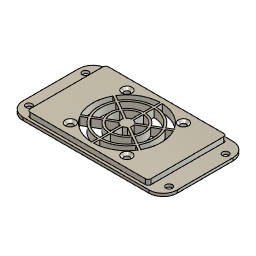
LCD cooling fan mod (Autodesk Fusion 360 design; units mm, degrees)
Autodesk Fusion 360 part; units mm, degrees
sketch "Sketch1" plane through (0, 0, 0) normal (0, 1, 0) x (1, 0, 0)
  line L0 (0, 0) -> (85.6, 0)
  line L1 (85.6, 0) -> (85.6, 55.5)
  line L2 (85.6, 55.5) -> (0, 55.5)
  line L3 (0, 55.5) -> (0, 0)
  line L4 (0, 55.5) -> (85.6, 0) construction
  line L5 (0, 0) -> (85.6, 55.5) construction
  line L6 (62.8, 47.75) -> (22.8, 47.75) construction
  line L7 (22.8, 47.75) -> (22.8, 7.75) construction
  line L8 (22.8, 7.75) -> (62.8, 7.75) construction
  line L9 (62.8, 7.75) -> (62.8, 47.75) construction
  line L10 (62.8, 47.75) -> (22.8, 7.75) construction
  line L11 (22.8, 47.75) -> (62.8, 7.75) construction
  circle A0 centre (62.8, 47.75) radius 1.9
  circle A1 centre (62.8, 7.75) radius 1.9
  circle A2 centre (22.8, 7.75) radius 1.9
  circle A3 centre (22.8, 47.75) radius 1.9
  line L12 (68.05, 2.5) -> (17.55, 2.5) construction
  line L13 (17.55, 2.5) -> (17.55, 53) construction
  line L14 (17.55, 53) -> (68.05, 53) construction
  line L15 (68.05, 53) -> (68.05, 2.5) construction
  line L16 (68.05, 2.5) -> (17.55, 53) construction
  line L17 (17.55, 2.5) -> (68.05, 53) construction
  circle A4 centre (42.8, 27.75) radius 24.25
  line L18 (43.55, 53) -> (42.05, 53) construction
  line L19 (42.05, 53) -> (42.05, 27.75)
  line L20 (42.05, 27.75) -> (43.55, 27.75)
  line L21 (43.55, 27.75) -> (43.55, 53)
  line L22 (43.175, 28.3995) -> (21.3079, 41.0245)
  line L23 (20.5579, 39.7255) -> (42.425, 27.1005)
  line L24 (42.425, 28.3995) -> (20.5579, 15.7745)
  line L25 (21.3079, 14.4755) -> (43.175, 27.1005)
  line L26 (42.05, 27.75) -> (42.05, 2.5)
  line L27 (43.55, 2.5) -> (43.55, 27.75)
  line L28 (42.425, 27.1005) -> (64.2921, 14.4755)
  line L29 (65.0421, 15.7745) -> (43.175, 28.3995)
  line L30 (43.175, 27.1005) -> (65.0421, 39.7255)
  line L31 (64.2921, 41.0245) -> (42.425, 28.3995)
  circle A5 centre (42.8, 27.75) radius 20
  circle A6 centre (42.8, 27.75) radius 18.5
  circle A7 centre (42.8, 27.75) radius 12.5
  circle A8 centre (42.8, 27.75) radius 11
  circle A9 centre (42.8, 27.75) radius 4
  line L32 (85.6, 7.25) -> (95.4, 7.25) construction
  circle A10 centre (93.15, 7.25) radius 2.25
  line L33 (93.15, 7.25) -> (93.15, 9.5) construction
  line L34 (93.15, 9.5) -> (93.15, 45) construction
  circle A11 centre (93.15, 47.25) radius 2.25
  line L35 (93.15, 47.25) -> (93.15, 45) construction
  line L36 (85.6, 0) -> (93.15, 0) construction
  line L37 (93.15, 0) -> (93.15, 7.25) construction
  line L38 (85.6, 7.25) -> (0, 7.25) construction
  line L39 (0, 7.25) -> (-6, 7.25) construction
  line L40 (-6, 7.25) -> (-6, 47.25) construction
  line L41 (93.15, 47.25) -> (-6, 47.25) construction
  circle A12 centre (-6, 47.25) radius 2.25
  circle A13 centre (-6, 7.25) radius 2.25
  line L42 (-11, 57.5) -> (98.15, 57.5)
  line L43 (98.15, 57.5) -> (98.15, -2)
  line L44 (98.15, -2) -> (-11, -2)
  line L45 (-11, -2) -> (-11, 57.5)
  point P0 (42.8, 27.75)
  point P1 (42.8, 27.75)
  dimension "d1" = 85.6
  dimension "d2" = 55.5
  dimension "d3" = 40
  dimension "d4" = 40
  dimension "d5" = 3.8
  dimension "d6" = 3.8
  dimension "d7" = 3.8
  dimension "d8" = 3.8
  dimension "d9" = 50.5
  dimension "d10" = 50.5
  dimension "d11" = 48.5
  dimension "d12" = 1.5
  dimension "d14" = 360
  dimension "d15" = -1.5
  dimension "d16" = 25
  dimension "d17" = -1.5
  dimension "d18" = 8
  dimension "d19" = 9.8
  dimension "d20" = 4.5
  dimension "d21" = 35.5
  dimension "d22" = 4.5
  dimension "d23" = 7.25
  dimension "d24" = 6
  dimension "d25" = 4.5
  dimension "d26" = 4.5
  dimension "d27" = 5
  dimension "d28" = 5
  dimension "d29" = 2
  dimension "d30" = 2
  constraint horizontal L0
  constraint vertical L1
  constraint horizontal L2
  constraint vertical L3
  constraint coincident L0.start L3.end
  constraint horizontal L6
  constraint perpendicular L6 L7
  constraint parallel L6 L8
  constraint parallel L7 L9
  constraint coincident L10 P1
  constraint coincident L11 P1
  constraint midpoint L5 P1
  constraint coincident L6.start L9.end
  constraint coincident L8.end L9.start
  constraint coincident L7.end L8.start
  constraint coincident L6.end L7.start
  constraint horizontal L12
  constraint perpendicular L12 L13
  constraint parallel L12 L14
  constraint parallel L13 L15
  constraint coincident L16 P1
  constraint coincident L17 P1
  constraint coincident P1 P0
  constraint horizontal L18
  constraint vertical L19
  constraint horizontal L20
  constraint vertical L21
  constraint midpoint L14 L18
  constraint midpoint P1 L20
  constraint tangent L9 A5
  constraint concentric A5 A9
  constraint coincident L1 L32.start
  constraint perpendicular L1 L32
  constraint coincident L32.end A10
  constraint coincident A10.centre L33.start
  constraint coincident A10 L33.end
  constraint perpendicular L32 L33
  constraint perpendicular L32 L34
  constraint coincident A11.centre L35.start
  constraint coincident A11 L34.end
  constraint vertical L35
  constraint coincident L34.end L35.end
  constraint coincident L32 A10.centre
  constraint perpendicular L1 L36
  constraint perpendicular L32 L37
  constraint coincident L3 L38.end
  constraint perpendicular L3 L38
  constraint perpendicular L3 L39
  constraint perpendicular L39 L40
  constraint perpendicular L35 L41
  constraint coincident L40 L41.end
  constraint coincident L40.end L41.end
  constraint coincident L39.end L40.start
  constraint horizontal L42
  constraint vertical L43
  constraint horizontal L44
  constraint vertical L45
  measures "d1" distance of L0.start L0.end
  measures "d2" distance of L0.start L2.end
  measures "d3" distance of L7.end L8.end
  measures "d4" distance of L6.end L7.end
  measures "d5" diameter of A0
  measures "d6" diameter of A1
  measures "d7" diameter of A2
  measures "d8" diameter of A3
  measures "d9" distance of L13.end L14.end
  measures "d10" distance of L12.end L13.end
  measures "d11" diameter of A4
  measures "d12" distance of L18.start L18.end
  measures "d16" diameter of A7
  measures "d18" diameter of A9
  measures "d19" distance of L32.start L32.end
  measures "d20" diameter of A10
  measures "d21" distance of L33.end L34.end
  measures "d22" diameter of A11
  measures "d23" distance of L36.end A10.centre
  measures "d24" distance of L38.end L39.end
  measures "d25" diameter of A12
  measures "d26" diameter of A13
  measures "d27" distance of L40.end L45
  measures "d28" distance of A11.centre L43
  measures "d29" distance of L2 L42
  measures "d30" distance of L0 L44
extrude "Extrude1" add sketch "Sketch1" along normal blind 3.6 and the other way blind 2 contours L0 L1 L2 L3 | A4 L30 L31 A5 | A4 L28 L29 A5 | L29 L30 A5 A6 | L30 L31 A5 A6 | L28 L29 A5 A6 | A4 L19 L21 A5 | L21 L31 A5 A6 | L30 L31 A6 A7 | A4 L26 L27 A5 | L27 L28 A5 A6 | L28 L29 A6 A7 | L19 L21 A5 A6 | L29 L30 A7 A8 | L30 L31 A7 A8 | L26 L27 A5 A6 | L28 L29 A7 A8 | A4 L22 L23 A5 | L19 L22 A5 A6 | L19 L21 A6 A7 | L21 L31 A7 A8 | L30 L31 A8 A9 | A4 L24 L25 A5 | L25 L26 A5 A6 | L26 L27 A6 A7 | L27 L28 A7 A8 | L28 L29 A8 A9 | L22 L23 A5 A6 | L19 L21 A7 A8 | L29 L30 A9 | L21 L29 L30 L31 A9 | L24 L25 A5 A6 | L26 L27 A7 A8 | L27 L28 L29 L30 A9 | L23 L24 A5 A6 | L22 L23 A6 A7 | L19 L22 A7 A8 | L19 L21 A8 A9 | L21 L31 A9 | L21 L27 L29 L30 | L24 L25 A6 A7 | L25 L26 A7 A8 | L26 L27 A8 A9 | L27 L28 A9 | L22 L23 A7 A8 | L19 L21 L22 L31 A9 | L21 L22 L29 L31 | L19 L20 L21 L22 L24 L29 L31 | L20 L23 L25 L26 L27 L28 L30 | L25 L27 L28 L30 | L24 L25 A7 A8 | L25 L26 L27 L28 A9 | L23 L24 A7 A8 | L22 L23 A8 A9 | L19 L22 A9 | L19 L22 L24 L31 | L24 L25 A8 A9 | L25 L26 A9 | L23 L25 L26 L28 | L19 L22 L23 L24 A9 | L19 L23 L24 L26 | L23 L24 L25 L26 A9 | L23 L24 A9
extrude "Extrude2" add sketch "Sketch1" against normal blind 2 contours L42 L43 L44 L45
fillet "Fillet1" radius 10 4 edges at (98.15, -1, -57.5) (98.15, -1, 2) (-11, -1, 2) (-11, -1, -57.5)
fillet "Fillet2" radius 2 4 edges at (0, 1.8, 0) (85.6, 1.8, 0) (85.6, 1.8, -55.5) (0, 1.8, -55.5)
chamfer "Chamfer1" distance 1.7 angle 45 4 edges at (21.0286, 3.6, -48.4371) (61.0286, 3.6, -48.4371) (61.0286, 3.6, -8.4371) (21.0286, 3.6, -8.4371)
